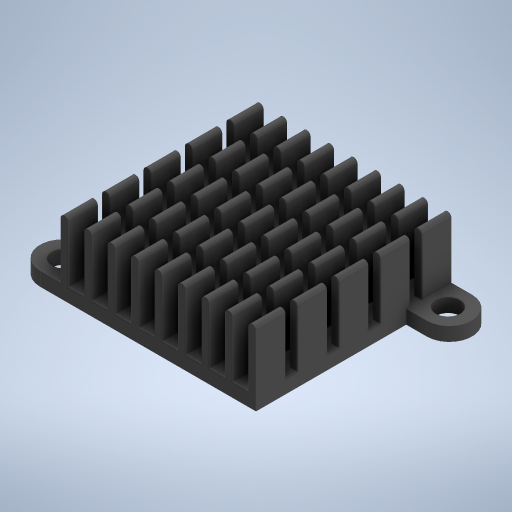
# Autodesk Inventor part: Heatsink-26x26x10-A
Saved by Autodesk Inventor 2024 (Build 280153000, 153)
## iProperties
Created: 2024-02-28
Part Number: Heatsink-26x26x10-A
Material: Generic
Document SubType Name: Modeling
Designer: danil
Density: 1 g/cm^3
Appearance: Default
Author: danil
Autodesk Inventor part; units mm, degrees
ref_plane "YZ Plane" through (0, 0, 0) normal (1, 0, 0) x (0, 1, 0)
ref_plane "XZ Plane" through (0, 0, 0) normal (0, 1, 0) x (-1, 0, 0)
ref_plane "XY Plane" through (0, 0, 0) normal (0, 0, 1) x (1, 0, 0)
sketch "Sketch1" plane through (0, 0, 0) normal (0, 1, 0) x (-1, 0, 0)
  line L0 (13, 13) -> (-13, 13)
  line L1 (-13, 13) -> (-13, -13)
  line L2 (-13, -13) -> (13, -13)
  line L3 (13, -13) -> (13, 13)
  line L4 (13, 13) -> (-13, -13) construction
  line L5 (-13, 13) -> (13, -13) construction
  line L6 (15.5644, 10) -> (-15.5644, -10) construction
  circle A0 centre (-15.5644, -10) radius 1.6
  line L7 (-13, -13) -> (-15.75, -13)
  line L8 (-13, -7) -> (-15.75, -7)
  line L9 (-15.75, -13) -> (-15.75, -7) construction
  arc A1 (-15.75, -7) -> (-15.75, -13) centre (-15.75, -10) ccw
  line L10 (0, -13) -> (0, 13) construction
  line L11 (13, 13) -> (15.75, 13)
  line L12 (13, 7) -> (15.75, 7)
  line L13 (15.75, 13) -> (15.75, 7) construction
  arc A2 (15.75, 7) -> (15.75, 13) centre (15.75, 10) ccw
  circle A3 centre (15.5644, 10) radius 1.6
  point P0 (0, 0)
  point P1 (-18.75, -10)
  point P2 (18.75, 10)
  dimension "d0" = 26
  dimension "d1" = 26
  dimension "d2" = 37
  dimension "d3" = 3.2
  dimension "d4" = 37.5
  dimension "d6" = 0.1856
  dimension "d7" = 6
  constraints: 28 end point, 8 midpoint, 6 point on circle, 5 horizontal, 4 centre point, 4 parallel, 2 coincident, 2 point on line, 2 vertical, 1 equal radius, 1 horizontal alignment, 1 perpendicular, 1 vertical alignment
  measures "d0" distance of L2.end L1.end
  measures "d1" distance of L1.end L0.end
  measures "d2" distance of L6.start L6.end
  measures "d3" diameter of A0
  measures "d4" horizontal distance of point (-18.75, -10) point (18.75, 10)
  measures "d6" distance of A1.centre L6.end
  measures "d7" distance between parallel lines of L8 L7
extrude "Extrusion1" add sketch "Sketch1" along normal blind 1.8
sketch "Sketch2" plane through (0, 1.8, 0) normal (0, 1, 0) x (1, 0, 0)
  line L0 (15.75, 13) -> (-13, 13) projected
  line L1 (-13, 13) -> (-12, 13)
  line L2 (-12, 13) -> (-12, 9.08)
  line L3 (-12, 9.08) -> (-13, 9.08)
  line L4 (-13, 9.08) -> (-13, 13)
  line L5 (-9.875, 13) -> (-8.875, 13)
  line L6 (-8.875, 13) -> (-8.875, 9.08)
  line L7 (-8.875, 9.08) -> (-9.875, 9.08)
  line L8 (-9.875, 9.08) -> (-9.875, 13)
  line L9 (-6.75, 13) -> (-5.75, 13)
  line L10 (-5.75, 13) -> (-5.75, 9.08)
  line L11 (-5.75, 9.08) -> (-6.75, 9.08)
  line L12 (-6.75, 9.08) -> (-6.75, 13)
  line L13 (-3.625, 13) -> (-2.625, 13)
  line L14 (-2.625, 13) -> (-2.625, 9.08)
  line L15 (-2.625, 9.08) -> (-3.625, 9.08)
  line L16 (-3.625, 9.08) -> (-3.625, 13)
  line L17 (-0.5, 13) -> (0.5, 13)
  line L18 (0.5, 13) -> (0.5, 9.08)
  line L19 (0.5, 9.08) -> (-0.5, 9.08)
  line L20 (-0.5, 9.08) -> (-0.5, 13)
  line L21 (2.625, 13) -> (3.625, 13)
  line L22 (3.625, 13) -> (3.625, 9.08)
  line L23 (3.625, 9.08) -> (2.625, 9.08)
  line L24 (2.625, 9.08) -> (2.625, 13)
  line L25 (5.75, 13) -> (6.75, 13)
  line L26 (6.75, 13) -> (6.75, 9.08)
  line L27 (6.75, 9.08) -> (5.75, 9.08)
  line L28 (5.75, 9.08) -> (5.75, 13)
  line L29 (8.875, 13) -> (9.875, 13)
  line L30 (9.875, 13) -> (9.875, 9.08)
  line L31 (9.875, 9.08) -> (8.875, 9.08)
  line L32 (8.875, 9.08) -> (8.875, 13)
  line L33 (12, 13) -> (13, 13)
  line L34 (13, 13) -> (13, 9.08)
  line L35 (13, 9.08) -> (12, 9.08)
  line L36 (12, 9.08) -> (12, 13)
  line L37 (-13, 7.48) -> (-12, 7.48)
  line L38 (-12, 7.48) -> (-12, 3.56)
  line L39 (-12, 3.56) -> (-13, 3.56)
  line L40 (-13, 3.56) -> (-13, 7.48)
  line L41 (-9.875, 7.48) -> (-8.875, 7.48)
  line L42 (-8.875, 7.48) -> (-8.875, 3.56)
  line L43 (-8.875, 3.56) -> (-9.875, 3.56)
  line L44 (-9.875, 3.56) -> (-9.875, 7.48)
  line L45 (-6.75, 7.48) -> (-5.75, 7.48)
  line L46 (-5.75, 7.48) -> (-5.75, 3.56)
  line L47 (-5.75, 3.56) -> (-6.75, 3.56)
  line L48 (-6.75, 3.56) -> (-6.75, 7.48)
  line L49 (-3.625, 7.48) -> (-2.625, 7.48)
  line L50 (-2.625, 7.48) -> (-2.625, 3.56)
  line L51 (-2.625, 3.56) -> (-3.625, 3.56)
  line L52 (-3.625, 3.56) -> (-3.625, 7.48)
  line L53 (-0.5, 7.48) -> (0.5, 7.48)
  line L54 (0.5, 7.48) -> (0.5, 3.56)
  line L55 (0.5, 3.56) -> (-0.5, 3.56)
  line L56 (-0.5, 3.56) -> (-0.5, 7.48)
  line L57 (2.625, 7.48) -> (3.625, 7.48)
  line L58 (3.625, 7.48) -> (3.625, 3.56)
  line L59 (3.625, 3.56) -> (2.625, 3.56)
  line L60 (2.625, 3.56) -> (2.625, 7.48)
  line L61 (5.75, 7.48) -> (6.75, 7.48)
  line L62 (6.75, 7.48) -> (6.75, 3.56)
  line L63 (6.75, 3.56) -> (5.75, 3.56)
  line L64 (5.75, 3.56) -> (5.75, 7.48)
  line L65 (8.875, 7.48) -> (9.875, 7.48)
  line L66 (9.875, 7.48) -> (9.875, 3.56)
  line L67 (9.875, 3.56) -> (8.875, 3.56)
  line L68 (8.875, 3.56) -> (8.875, 7.48)
  line L69 (12, 7.48) -> (13, 7.48)
  line L70 (13, 7.48) -> (13, 3.56)
  line L71 (13, 3.56) -> (12, 3.56)
  line L72 (12, 3.56) -> (12, 7.48)
  line L73 (-13, 1.96) -> (-12, 1.96)
  line L74 (-12, 1.96) -> (-12, -1.96)
  line L75 (-12, -1.96) -> (-13, -1.96)
  line L76 (-13, -1.96) -> (-13, 1.96)
  line L77 (-9.875, 1.96) -> (-8.875, 1.96)
  line L78 (-8.875, 1.96) -> (-8.875, -1.96)
  line L79 (-8.875, -1.96) -> (-9.875, -1.96)
  line L80 (-9.875, -1.96) -> (-9.875, 1.96)
  line L81 (-6.75, 1.96) -> (-5.75, 1.96)
  line L82 (-5.75, 1.96) -> (-5.75, -1.96)
  line L83 (-5.75, -1.96) -> (-6.75, -1.96)
  line L84 (-6.75, -1.96) -> (-6.75, 1.96)
  line L85 (-3.625, 1.96) -> (-2.625, 1.96)
  line L86 (-2.625, 1.96) -> (-2.625, -1.96)
  line L87 (-2.625, -1.96) -> (-3.625, -1.96)
  line L88 (-3.625, -1.96) -> (-3.625, 1.96)
  line L89 (-0.5, 1.96) -> (0.5, 1.96)
  line L90 (0.5, 1.96) -> (0.5, -1.96)
  line L91 (0.5, -1.96) -> (-0.5, -1.96)
  line L92 (-0.5, -1.96) -> (-0.5, 1.96)
  line L93 (2.625, 1.96) -> (3.625, 1.96)
  line L94 (3.625, 1.96) -> (3.625, -1.96)
  line L95 (3.625, -1.96) -> (2.625, -1.96)
  line L96 (2.625, -1.96) -> (2.625, 1.96)
  line L97 (5.75, 1.96) -> (6.75, 1.96)
  line L98 (6.75, 1.96) -> (6.75, -1.96)
  line L99 (6.75, -1.96) -> (5.75, -1.96)
  line L100 (5.75, -1.96) -> (5.75, 1.96)
  line L101 (8.875, 1.96) -> (9.875, 1.96)
  line L102 (9.875, 1.96) -> (9.875, -1.96)
  line L103 (9.875, -1.96) -> (8.875, -1.96)
  line L104 (8.875, -1.96) -> (8.875, 1.96)
  line L105 (12, 1.96) -> (13, 1.96)
  line L106 (13, 1.96) -> (13, -1.96)
  line L107 (13, -1.96) -> (12, -1.96)
  line L108 (12, -1.96) -> (12, 1.96)
  line L109 (-13, -3.56) -> (-12, -3.56)
  line L110 (-12, -3.56) -> (-12, -7.48)
  line L111 (-12, -7.48) -> (-13, -7.48)
  line L112 (-13, -7.48) -> (-13, -3.56)
  line L113 (-9.875, -3.56) -> (-8.875, -3.56)
  line L114 (-8.875, -3.56) -> (-8.875, -7.48)
  line L115 (-8.875, -7.48) -> (-9.875, -7.48)
  line L116 (-9.875, -7.48) -> (-9.875, -3.56)
  line L117 (-6.75, -3.56) -> (-5.75, -3.56)
  line L118 (-5.75, -3.56) -> (-5.75, -7.48)
  line L119 (-5.75, -7.48) -> (-6.75, -7.48)
  line L120 (-6.75, -7.48) -> (-6.75, -3.56)
  line L121 (-3.625, -3.56) -> (-2.625, -3.56)
  line L122 (-2.625, -3.56) -> (-2.625, -7.48)
  line L123 (-2.625, -7.48) -> (-3.625, -7.48)
  line L124 (-3.625, -7.48) -> (-3.625, -3.56)
  line L125 (-0.5, -3.56) -> (0.5, -3.56)
  line L126 (0.5, -3.56) -> (0.5, -7.48)
  line L127 (0.5, -7.48) -> (-0.5, -7.48)
  line L128 (-0.5, -7.48) -> (-0.5, -3.56)
  line L129 (2.625, -3.56) -> (3.625, -3.56)
  line L130 (3.625, -3.56) -> (3.625, -7.48)
  line L131 (3.625, -7.48) -> (2.625, -7.48)
  line L132 (2.625, -7.48) -> (2.625, -3.56)
  line L133 (5.75, -3.56) -> (6.75, -3.56)
  line L134 (6.75, -3.56) -> (6.75, -7.48)
  line L135 (6.75, -7.48) -> (5.75, -7.48)
  line L136 (5.75, -7.48) -> (5.75, -3.56)
  line L137 (8.875, -3.56) -> (9.875, -3.56)
  line L138 (9.875, -3.56) -> (9.875, -7.48)
  line L139 (9.875, -7.48) -> (8.875, -7.48)
  line L140 (8.875, -7.48) -> (8.875, -3.56)
  line L141 (12, -3.56) -> (13, -3.56)
  line L142 (13, -3.56) -> (13, -7.48)
  line L143 (13, -7.48) -> (12, -7.48)
  line L144 (12, -7.48) -> (12, -3.56)
  line L145 (-13, -9.08) -> (-12, -9.08)
  line L146 (-12, -9.08) -> (-12, -13)
  line L147 (-12, -13) -> (-13, -13)
  line L148 (-13, -13) -> (-13, -9.08)
  line L149 (-9.875, -9.08) -> (-8.875, -9.08)
  line L150 (-8.875, -9.08) -> (-8.875, -13)
  line L151 (-8.875, -13) -> (-9.875, -13)
  line L152 (-9.875, -13) -> (-9.875, -9.08)
  line L153 (-6.75, -9.08) -> (-5.75, -9.08)
  line L154 (-5.75, -9.08) -> (-5.75, -13)
  line L155 (-5.75, -13) -> (-6.75, -13)
  line L156 (-6.75, -13) -> (-6.75, -9.08)
  line L157 (-3.625, -9.08) -> (-2.625, -9.08)
  line L158 (-2.625, -9.08) -> (-2.625, -13)
  line L159 (-2.625, -13) -> (-3.625, -13)
  line L160 (-3.625, -13) -> (-3.625, -9.08)
  line L161 (-0.5, -9.08) -> (0.5, -9.08)
  line L162 (0.5, -9.08) -> (0.5, -13)
  line L163 (0.5, -13) -> (-0.5, -13)
  line L164 (-0.5, -13) -> (-0.5, -9.08)
  line L165 (2.625, -9.08) -> (3.625, -9.08)
  line L166 (3.625, -9.08) -> (3.625, -13)
  line L167 (3.625, -13) -> (2.625, -13)
  line L168 (2.625, -13) -> (2.625, -9.08)
  line L169 (5.75, -9.08) -> (6.75, -9.08)
  line L170 (6.75, -9.08) -> (6.75, -13)
  line L171 (6.75, -13) -> (5.75, -13)
  line L172 (5.75, -13) -> (5.75, -9.08)
  line L173 (8.875, -9.08) -> (9.875, -9.08)
  line L174 (9.875, -9.08) -> (9.875, -13)
  line L175 (9.875, -13) -> (8.875, -13)
  line L176 (8.875, -13) -> (8.875, -9.08)
  line L177 (12, -9.08) -> (13, -9.08)
  line L178 (13, -9.08) -> (13, -13)
  line L179 (13, -13) -> (12, -13)
  line L180 (12, -13) -> (12, -9.08)
  point P0 (0, 0)
  dimension "d10" = 1
  dimension "d11" = 3.92
  dimension "d14" = 3.125
  dimension "d17" = 5.52
  constraints: 360 end point, 2 horizontal, 2 parallel, 1 collinear, 1 perpendicular, 1 vertical, 351 other
  measures "d10" distance of L2.end L3.end
  measures "d11" distance of L1.end L2.end
  measures "d14" distance of L0.end L5.start
  measures "d17" distance of L0.end L37.start
extrude "Extrusion2" add sketch "Sketch2" along normal blind 8
fillet "Fillet1" radius 0.5 50 edges at (-12, 9.8, 0) (-12, 9.8, -5.52) (-12, 9.8, -11.04) (-12, 9.8, 5.52) (-12, 9.8, 11.04) (-13, 9.8, 0) (-13, 9.8, -5.52) (-13, 9.8, -11.04) (-13, 9.8, 5.52) (-13, 9.8, 11.04) (-9.875, 9.8, 0) (-9.875, 9.8, 5.52) (-9.875, 9.8, -5.52) (-9.875, 9.8, -11.04) (-9.875, 9.8, 11.04) (-8.875, 9.8, 5.52) (-8.875, 9.8, 0) (-8.875, 9.8, -5.52) (-8.875, 9.8, 11.04) (-8.875, 9.8, -11.04) (-6.75, 9.8, 11.04) (-6.75, 9.8, 5.52) (-6.75, 9.8, 0) (-6.75, 9.8, -5.52) (-6.75, 9.8, -11.04) (-5.75, 9.8, 5.52) (-5.75, 9.8, 11.04) (-5.75, 9.8, -11.04) (-5.75, 9.8, 0) (-5.75, 9.8, -5.52) (-3.625, 9.8, 0) (-3.625, 9.8, -5.52) (-3.625, 9.8, 5.52) (-3.625, 9.8, -11.04) (-3.625, 9.8, 11.04) (-2.625, 9.8, -5.52) (-2.625, 9.8, 5.52) (-2.625, 9.8, -11.04) (-2.625, 9.8, 0) (-2.625, 9.8, 11.04) (-0.5, 9.8, 11.04) (-0.5, 9.8, 0) (-0.5, 9.8, -11.04) (-0.5, 9.8, 5.52) (-0.5, 9.8, -5.52) (0.5, 9.8, 11.04) (0.5, 9.8, -11.04) (0.5, 9.8, 5.52) (0.5, 9.8, -5.52) (0.5, 9.8, 0)
fillet "Fillet2" radius 0.5 40 edges at (2.625, 9.8, 0) (2.625, 9.8, -5.52) (2.625, 9.8, 5.52) (2.625, 9.8, -11.04) (2.625, 9.8, 11.04) (3.625, 9.8, 0) (3.625, 9.8, -5.52) (3.625, 9.8, 5.52) (3.625, 9.8, -11.04) (3.625, 9.8, 11.04) (5.75, 9.8, -5.52) (5.75, 9.8, 0) (5.75, 9.8, 11.04) (5.75, 9.8, 5.52) (5.75, 9.8, -11.04) (6.75, 9.8, 5.52) (6.75, 9.8, 0) (6.75, 9.8, 11.04) (6.75, 9.8, -5.52) (6.75, 9.8, -11.04) (8.875, 9.8, -5.52) (8.875, 9.8, 5.52) (8.875, 9.8, 11.04) (8.875, 9.8, 0) (8.875, 9.8, -11.04) (9.875, 9.8, -5.52) (9.875, 9.8, 5.52) (9.875, 9.8, 11.04) (9.875, 9.8, 0) (9.875, 9.8, -11.04) (12, 9.8, 11.04) (12, 9.8, 0) (12, 9.8, 5.52) (12, 9.8, -5.52) (12, 9.8, -11.04) (13, 9.8, 11.04) (13, 9.8, 0) (13, 9.8, -11.04) (13, 9.8, 5.52) (13, 9.8, -5.52)
body "Solid1"
